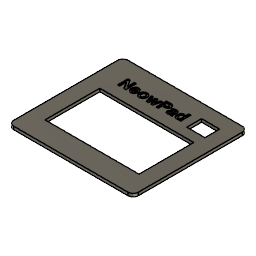
Top (Autodesk Fusion 360 design; units mm, degrees)
part number: 2026-03-31-19-46-04-300
Autodesk Fusion 360 part; units mm, degrees
sketch "Boceto1" plane through (0, 0, 0) normal (0, 0, 1) x (1, 0, 0)
  line L0 (60.5, -55.5) -> (-60.5, -55.5)
  line L1 (-60.5, -55.5) -> (-60.5, 55.5)
  line L2 (-60.5, 55.5) -> (60.5, 55.5)
  line L3 (60.5, 55.5) -> (60.5, -55.5)
  line L4 (60.5, -55.5) -> (-60.5, 55.5) construction
  line L5 (-60.5, -55.5) -> (60.5, 55.5) construction
  line L6 (50.5, -45.5) -> (-50.5, 45.5) construction
  line L7 (-50.5, -45.5) -> (50.5, 45.5) construction
  line L8 (-50.5, -45.5) -> (-45.585, -45.5)
  line L9 (-45.585, -34.875) -> (-50.5, -34.875)
  line L10 (-50.5, -34.875) -> (-50.5, -45.5)
  line L11 (50.5, -45.5) -> (45.585, -45.5)
  line L12 (45.585, -34.875) -> (50.5, -34.875)
  line L13 (50.5, -34.875) -> (50.5, -45.5)
  line L14 (-45.585, -34.875) -> (45.585, -34.875)
  line L15 (45.585, -34.875) -> (45.585, 18.195)
  line L16 (45.585, 18.195) -> (-45.585, 18.195)
  line L17 (-45.585, 18.195) -> (-45.585, -34.875)
  line L18 (50.5, 45.5) -> (46.85, 45.5)
  line L19 (46.85, 41.98) -> (50.5, 41.98)
  line L20 (50.5, 41.98) -> (50.5, 45.5)
  line L21 (46.85, 41.98) -> (29.35, 41.98)
  line L22 (29.35, 41.98) -> (29.35, 27.78)
  line L23 (29.35, 27.78) -> (46.85, 27.78)
  line L24 (46.85, 27.78) -> (46.85, 41.98)
  dimension "d1" = 121
  dimension "d2" = 111
  dimension "d3" = 101
  dimension "d4" = 91
  dimension "d5" = 4.915
  dimension "d6" = 10.625
  dimension "d7" = 4.915
  dimension "d8" = 10.625
  dimension "d10" = 53.07
  dimension "d11" = 3.65
  dimension "d12" = 3.52
  dimension "d13" = 17.5
  dimension "d14" = 14.2
  constraint horizontal L0
  constraint perpendicular L0 L1
  constraint parallel L0 L2
  constraint parallel L1 L3
  constraint coincident L4 origin
  constraint coincident L5 origin
  constraint coincident L6 origin
  constraint coincident L7 origin
  constraint horizontal L8
  constraint horizontal L9
  constraint vertical L10
  constraint horizontal L11
  constraint horizontal L12
  constraint vertical L13
  constraint horizontal L14
  constraint vertical L15
  constraint horizontal L16
  constraint vertical L17
  constraint horizontal L18
  constraint horizontal L19
  constraint vertical L20
  constraint horizontal L21
  constraint vertical L22
  constraint horizontal L23
  constraint vertical L24
  measures "d1" distance of L1.end L2.end
  measures "d2" distance of L0.end L1.end
  measures "d3" distance of L6.end L7.end
  measures "d4" distance of L7.start L6.end
  measures "d5" distance of L7.start L8.end
  measures "d6" distance of L7.start L9.end
  measures "d7" distance of L6.start L11.end
  measures "d8" distance of L6.start L12.end
  measures "d10" distance of L9.start L16.end
  measures "d11" distance of L7.end L18.end
  measures "d12" distance of L7.end L19.end
  measures "d13" distance of L19.start L21.end
  measures "d14" distance of L19.start L23.end
extrude "Extruir1" add sketch "Boceto1" along normal blind 3
sketch "Boceto2" plane through (0, 0, 3) normal (0, 0, 1) x (-1, 0, 0)
  line L0 (-46.85, -41.98) -> (-46.85, -27.78)
  line L1 (-46.85, -27.78) -> (-29.35, -27.78)
  line L2 (-29.35, -27.78) -> (-29.35, -41.98)
  line L3 (-29.35, -41.98) -> (-46.85, -41.98)
  line L4 (45.585, 34.875) -> (45.585, -18.195)
  line L5 (45.585, -18.195) -> (-45.585, -18.195)
  line L6 (-45.585, -18.195) -> (-45.585, 34.875)
  line L7 (-45.585, 34.875) -> (45.585, 34.875)
  line L8 (-60.5, -55.5) -> (60.5, -55.5)
  line L9 (60.5, -55.5) -> (60.5, 55.5)
  line L10 (60.5, 55.5) -> (-60.5, 55.5)
  line L11 (-60.5, 55.5) -> (-60.5, -55.5)
  line L12 (27.0674, -28.1508) -> (-8.5281, -28.1508) construction
  line L13 (-8.5281, -28.1508) -> (-8.5281, -41.528) construction
  line L14 (-8.5281, -41.528) -> (27.0674, -41.528) construction
  line L15 (27.0674, -41.528) -> (27.0674, -28.1508) construction
  dimension "d17" = 10
  text T0 "NeowPad" font "Arial" height 10 bold align centre middle in box 35.5954 x 13.3772 at (27.0674, -28.1508) x (-1, 0) y (0, -1) spacing 1
extrude "Extruir2" cut sketch "Boceto2" against normal blind 1 text T0
move_body "Desplazar1" bodies 1 to x (1, 0, 0) y (0, 1, 0) z (0, 0, 1) at (0, 0, -5)
fillet "Empalme1" radius 5 4 edges at (-60.5, -55.5, -3.5) (-60.5, 55.5, -3.5) (60.5, 55.5, -3.5) (60.5, -55.5, -3.5)
equation "d1 = 100 mm + 1 mm + 20 mm"
equation "d2 = 90 mm + 1 mm + 20 mm"
equation "d3 = 100 mm + 1 mm"
equation "d4 = 90 mm + 1 mm"
equation "d11 = 3.15 mm + 0.5 mm"
equation "d12 = 3.02 mm + 0.5 mm"
equation "d18 = 'NeowPad'"
